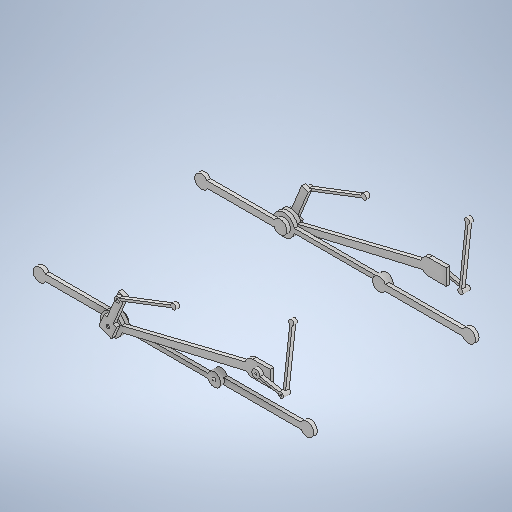
# Autodesk Inventor part: Linkage Arms [Copy]
Saved by Autodesk Inventor 2025.1 (Build 291241020, 241B)
## iProperties
Created: 2022-11-28
Part Number: Linkage Arms [Copy]
Material: Generic
Document SubType Name: Modeling
Designer: mc_vlongo24
Density: 1 g/cm^3
Appearance: Default
Author: mc_vlongo24
Autodesk Inventor part; units mm, degrees
sketch "Sketch1" plane through (0, 0, 0) normal (0, 0, 1) x (1, 0, 0)
  circle A0 centre (-1.5499, -0.0498) radius 2.3876
  circle A1 centre (-33.1609, 0) radius 2.3813
  line L0 (-31.002, 1.0048) -> (-3.692, 1.0048)
  line L1 (-31.1066, -1.2043) -> (-3.6398, -1.2043)
  dimension "d0" = 4.7752
  dimension "d1" = 4.7625
  constraints: 4 end point, 4 point on circle, 2 centre point, 1 coincident, 1 horizontal, 1 parallel
  measures "d0" diameter of A0
  measures "d1" diameter of A1
extrude "Extrusion1" add sketch "Sketch1" along normal blind 1.27
ref_plane "Work Plane3" through (0, 0, 2.54) normal (0, 0, 1) x (1, 0, 0)
sketch "Sketch3" plane through (0, 0, 2.54) normal (0, 0, 1) x (1, 0, 0)
  arc A0 (-64.4126, 0.3327) -> (-64.704, -1.4958) centre (-68.208, 0) ccw projected
  circle A1 centre (-68.208, 0) radius 3.81
  circle A2 centre (-18.2102, 11.4321) radius 2.8575
  line L0 (-18.2058, 14.2896) -> (-11.9889, 14.28)
  line L1 (-18.2146, 8.5746) -> (-11.9977, 8.565)
  line L2 (-11.9977, 8.565) -> (-11.9889, 14.28)
  line L3 (-64.4588, -0.6776) -> (-20.3903, 9.5847)
  line L4 (-64.6471, 1.3549) -> (-20.9742, 12.1572)
  point P0 (0, 0)
  point P1 (-64.704, -1.4958)
  point P2 (-64.6471, 1.3549)
  point P3 (-64.4126, 0.3327)
  dimension "d9" = 5.715
  constraints: 10 end point, 6 point on circle, 2 centre point, 2 perpendicular, 2 tangent, 1 coincident
  measures "d9" diameter of A2
extrude "Extrusion3" add sketch "Sketch3" along normal blind 1.27 contours A0 L4 A2 L3 A1 | A2 | L0 L2 L1 A2
sketch "Sketch4" plane through (0, 0, 3.81) normal (0, 0, 1) x (1, 0, 0)
  line L0 (-69.5113, 3.0309) -> (-71.3364, -1.3818)
  line L1 (-71.3364, -1.3818) -> (-66.9355, -3.202)
  line L2 (-66.9355, -3.202) -> (-65.1104, 1.2106)
  line L3 (-65.1104, 1.2106) -> (-69.5113, 3.0309)
  line L4 (-68.5325, 2.626) -> (-64.3854, 12.653)
  line L5 (-64.3854, 12.653) -> (-62.1347, 11.7221)
  line L6 (-62.1347, 11.7221) -> (-66.2818, 1.6951)
  point P0 (0, 0)
  dimension "d12" = 4.7752
  dimension "d13" = 4.7625
  constraints: 14 end point, 5 parallel, 2 point on line
  measures "d12" distance between parallel lines of L1 L3
  measures "d13" distance between parallel lines of L2 L0
extrude "Extrusion4" add sketch "Sketch4" along normal blind 1.27
sketch "Sketch5" plane through (0, 0, 5.08) normal (0, 0, 1) x (1, 0, 0)
  circle A0 centre (-63.5763, 11.1153) radius 0.9525
  line L0 (-63.0163, 11.8857) -> (-43.8623, 19.2371)
  line L1 (-43.8623, 19.2371) -> (-43.6057, 18.5447)
  line L2 (-43.6057, 18.5447) -> (-64.3629, 10.5781)
  circle A1 centre (-43.734, 18.8909) radius 0.9525
  point P0 (0, 0)
  point P1 (-44.4215, 18.2316)
  point P2 (-44.686, 18.9209)
  point P3 (-62.6323, 11.2422)
  dimension "d16" = 1.905
  dimension "d17" = 1.905
  constraints: 6 end point, 2 centre point, 2 point on circle, 1 midpoint, 1 parallel
  measures "d16" diameter of A0
  measures "d17" diameter of A1
extrude "Extrusion5" add sketch "Sketch5" along normal blind 1.27
ref_plane "Work Plane2" through (0, 0, 1.27) normal (0, 0, -1) x (-1, 0, 0)
sketch "Sketch6" plane through (0, 0, 1.27) normal (0, 0, -1) x (-1, 0, 0)
  arc A0 (65.7715, 2.9291) -> (68.0442, 3.8065) centre (68.208, 0) ccw projected
  circle A1 centre (68.208, 0) radius 2.3876
  circle A2 centre (96.0964, -0.0556) radius 2.3812
  line L0 (70.3193, -1.1149) -> (93.9638, -1.1149)
  line L1 (70.2674, 1.2082) -> (94.0782, 1.2082)
  point P0 (0, 0)
  point P1 (64.4588, -0.6776)
  point P2 (71.8214, 1.2082)
  point P3 (71.8513, -1.1149)
  point P4 (64.6471, 1.3549)
  dimension "d20" = 4.7752
  dimension "d21" = 4.7625
  constraints: 4 end point, 4 point on circle, 2 centre point, 1 coincident, 1 horizontal, 1 parallel
  measures "d20" diameter of A1
  measures "d21" diameter of A2
extrude "Extrusion6" add sketch "Sketch6" along normal blind 1.27
sketch "Sketch7" plane through (0, 0, 3.81) normal (0, 0, 1) x (1, 0, 0)
  circle A0 centre (-15.8608, 11.6095) radius 1.4351
  circle A1 centre (-7.005, 9.5359) radius 0.9525
  line L0 (-14.431, 11.4858) -> (-7.6964, 10.1909)
  line L1 (-14.7048, 10.759) -> (-7.9545, 9.4611)
  point P0 (0, 0)
  dimension "d25" = 2.8702
  dimension "d26" = 1.905
  dimension "d34" = 0.7654
  constraints: 4 end point, 4 point on circle, 2 centre point, 1 parallel
  measures "d25" diameter of A0
  measures "d26" diameter of A1
  measures "d34" distance between parallel lines of L0 L1
extrude "Extrusion7" add sketch "Sketch7" along normal blind 1.27
sketch "Sketch8" plane through (0, 0, 3.81) normal (0, 0, -1) x (-1, 0, 0)
  arc A0 (7.6964, 10.1909) -> (7.9545, 9.4611) centre (7.005, 9.5359) ccw projected
  circle A1 centre (7.005, 9.5359) radius 0.9525
  circle A2 centre (4.6234, 32.3514) radius 0.9525
  line L0 (4.3076, 31.4528) -> (6.5893, 10.3929)
  line L1 (7.4206, 10.3929) -> (5.129, 31.5442)
  point P0 (0, 0)
  point P1 (7.4206, 10.3929)
  dimension "d29" = 1.905
  constraints: 4 end point, 4 point on circle, 2 centre point, 1 coincident, 1 parallel
  measures "d29" diameter of A2
extrude "Extrusion8" add sketch "Sketch8" along normal blind 1.27
ref_plane "Work Plane1" through (0, 0, -27.94) normal (0, 0, -1) x (-1, 0, 0)
extrude "Extrusion9" add sketch "Sketch3" along normal blind 1.27
sketch "Sketch9" plane through (0, 0, 1.27) normal (0, 0, 1) x (1, 0, 0)
  arc A0 (-31.2983, 1.4836) -> (-31.2983, -1.4836) centre (-33.1609, 0) ccw projected
  circle A1 centre (-33.1609, 0) radius 2.3813
  circle A2 centre (-68.195, -0.0041) radius 3.81
  line L0 (-35.4136, -0.7718) -> (-64.4631, -0.7718)
  line L1 (-64.4648, 0.7718) -> (-35.4136, 0.7718)
  point P0 (0, 0)
  point P1 (-31.2983, -1.4836)
  point P2 (-31.2983, 1.4836)
  dimension "d37" = 7.62
  constraints: 4 end point, 4 point on circle, 2 centre point, 1 coincident, 1 horizontal, 1 parallel
  measures "d37" diameter of A2
extrude "Extrusion10" add sketch "Sketch9" along normal blind 1.27
sketch "Sketch11" plane through (0, 0, 2.54) normal (0, 0, 1) x (1, 0, 0)
  arc A0 (-31.1066, -1.2043) -> (-31.002, 1.0048) centre (-33.1609, 0) ccw projected
  circle A1 centre (-33.1609, 0) radius 0.635
  point P0 (0, 0)
  dimension "d43" = 1.27
  constraints: 1 centre point, 1 coincident
  measures "d43" diameter of A1
extrude "Extrusion12" add sketch "Sketch11" along normal blind 0.508 and the other way blind 2.54
sketch "Sketch12" plane through (0, 0, 0) normal (0, 0, -1) x (-1, 0, 0)
  circle A0 centre (68.208, 0) radius 3.81 projected
  circle A1 centre (68.208, 0) radius 0.635
  point P0 (0, 0)
  dimension "d48" = 1.27
  constraints: 1 centre point, 1 coincident
  measures "d48" diameter of A1
extrude "Extrusion13" add sketch "Sketch12" along normal blind 0.0254 and the other way blind 5.334 contours A1
sketch "Sketch13" plane through (0, 0, 6.35) normal (0, 0, 1) x (1, 0, 0)
  arc A0 (-63.0163, 11.8857) -> (-62.6323, 11.2422) centre (-63.5763, 11.1153) ccw projected
  circle A1 centre (-63.5763, 11.1153) radius 0.3175
  point P0 (0, 0)
  dimension "d53" = 0.635
  constraints: 1 centre point, 1 coincident
  measures "d53" diameter of A1
extrude "Extrusion14" add sketch "Sketch13" along normal blind 0.254 and the other way blind 2.54
sketch "Sketch14" plane through (0, 0, 5.08) normal (0, 0, 1) x (1, 0, 0)
  arc A0 (-14.431, 11.4858) -> (-14.7048, 10.759) centre (-15.8608, 11.6095) ccw projected
  circle A1 centre (-15.8608, 11.6095) radius 0.3175
  arc A2 (-7.9545, 9.4611) -> (-7.6964, 10.1909) centre (-7.005, 9.5359) ccw projected
  circle A3 centre (-7.005, 9.5359) radius 0.3175
  point P0 (0, 0)
  dimension "d58" = 0.635
  dimension "d59" = 0.635
  constraints: 2 centre point, 2 coincident
  measures "d58" diameter of A1
  measures "d59" diameter of A3
extrude "Extrusion15" add sketch "Sketch14" along normal blind 0.254 and the other way blind 2.54
fillet "Fillet3" radius 0.254 4 edges at (-67.573, 0, 5.334) (-7.3225, 9.5359, 5.334) (-16.1783, 11.6095, 5.334) (-63.8938, 11.1153, 6.604)
fillet "Fillet4" radius 0.508 1 edges at (-33.7959, 0, 3.048)
mirror "Mirror2" about plane through (0, 0, -27.94) normal (0, 0, -1) of "Extrusion6", "Extrusion4", "Extrusion3", "Extrusion10", "Extrusion9", "Extrusion5", "Extrusion1", "Extrusion7", "Extrusion8"
sketch "Sketch15" plane through (-68.5325, 2.626, -60.96) normal (0, 0, -1) x (-0.9240806, 0.3821977, 0)
  circle A0 centre (-1.3035, -2.3026) radius 0.381 projected
  circle A1 centre (-1.3035, -2.3026) radius 0.635
  point P0 (-64.3332, 23.7663)
  constraints: 1 centre point, 1 coincident
extrude "Extrusion16" add sketch "Sketch15" along normal blind 0.254 and the other way blind 5.08 contours A0 | A1
sketch "Sketch16" plane through (-44.686, 18.9209, -62.23) normal (0, 0, -1) x (-0.9335991, -0.3583192, 0)
  circle A0 centre (20.4329, -0.5186) radius 0.0635 projected
  circle A1 centre (20.4329, -0.5186) radius 0.3175
  point P0 (-34.9391, -33.6764)
  constraints: 1 centre point, 1 coincident
extrude "Extrusion17" add sketch "Sketch16" along normal blind 0.254 and the other way blind 2.54 contours A0 | A1
sketch "Sketch17" plane through (-35.4136, -0.7718, -58.42) normal (0, 0, -1) x (-1, 0, 0)
  circle A0 centre (-2.2527, 0.7718) radius 0.127 projected
  circle A1 centre (-2.2527, 0.7718) radius 0.635
  point P0 (-35.4136, 0.7718)
  constraints: 1 centre point, 1 coincident
extrude "Extrusion18" add sketch "Sketch17" along normal blind 0.254 and the other way blind 2.54 contours A0 | A1
sketch "Sketch18" plane through (-15.8608, 11.6095, -60.96) normal (0, 0, -1) x (-0.9357807, 0.3525825, 0)
  circle A0 centre (0, 0) radius 0.0635 projected
  circle A1 centre (0, 0) radius 0.3175
  circle A2 centre (-9.0182, 1.1819) radius 0.0635 projected
  circle A3 centre (-9.0182, 1.1819) radius 0.3175
  point P0 (-18.9355, -5.2718)
  constraints: 2 centre point, 2 coincident
extrude "Extrusion19" add sketch "Sketch18" along normal blind 0.254 and the other way blind 2.54 contours A0 | A1 | A2 | A3
fillet "Fillet5" radius 0.254 5 edges at (-32.5259, 0, -58.674) (-67.6213, -0.2426, -61.214) (-6.7078, 9.4239, -61.214) (-63.2799, 11.229, -62.484) (-15.5636, 11.4976, -61.214)
body "Solid1"
